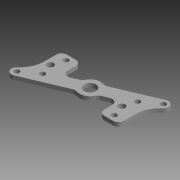
# Autodesk Inventor part: 01105
Saved by Autodesk Inventor 2015 (Build 190159000, 159)
## iProperties
Created: 2015-09-02
Part Number: 01105
Material: Generic
Description: Spring holder plate
Document SubType Name: Modeling
Designer: FC
Density: 1 g/cm^3
Appearance: Default
Part Category: 5 - Engine
Author: francis
Autodesk Inventor part; units mm, degrees
ref_plane "YZ Plane" through (0, 0, 0) normal (1, 0, 0) x (0, 1, 0)
ref_plane "XY Plane" through (0, 0, 0) normal (0, 0, 1) x (1, 0, 0)
sketch "Sketch1" plane through (0, 0, 0) normal (0, 0, 1) x (1, 0, 0)
  circle A0 centre (-10.5, 0) radius 2.067 construction
  circle A1 centre (-7.5, -9) radius 1.7295 construction
  circle A2 centre (-7.5, 9) radius 1.7295 construction
  circle A3 centre (-7.5, 9) radius 1.7295 construction
  circle A4 centre (-7.5, -9) radius 1.7295 construction
  circle A5 centre (-10.5, 0) radius 2.067 construction
  line L0 (0, -13) -> (-15, -13) construction
  line L1 (0, 13) -> (0, -13) construction
  line L2 (-15, 13) -> (0, 13) construction
  line L3 (-15, -13) -> (-15, 13) construction
  circle A6 centre (-62.5, -9) radius 1.7295 construction
  circle A7 centre (-62.5, 9) radius 1.7295 construction
  circle A8 centre (-65.5, 0) radius 2.067 construction
  line L4 (-55, -13) -> (-70, -13) construction
  line L5 (-55, 13) -> (-55, -13) construction
  line L6 (-70, 13) -> (-55, 13) construction
  line L7 (-70, -13) -> (-70, 13) construction
  spline S0 degree 3 poles (-35, 4) (-35.5054, 4) (-36.0423, 3.8984) (-37.0269, 3.4894) (-37.4748, 3.182) (-38.1819, 2.4749) (-38.4894, 2.027) (-38.8985, 1.0423) (-39, 0.5052) (-39, -0.5052) (-38.8985, -1.0423) (-38.4894, -2.027) (-38.1819, -2.4749) (-37.4748, -3.182) (-37.0269, -3.4894) (-36.0423, -3.8984) (-35.5054, -4) (-34.4946, -4) (-33.9577, -3.8984) (-32.9731, -3.4894) (-32.5252, -3.182) (-31.8181, -2.4749) (-31.5106, -2.027) (-31.1015, -1.0423) (-31, -0.5052) (-31, 0.5052) (-31.1015, 1.0423) (-31.5106, 2.027) (-31.8181, 2.4749) (-32.5252, 3.182) (-32.9731, 3.4894) (-33.9577, 3.8984) (-34.4946, 4) (-35, 4) knots 0 0 0 0 0.151609 0.151609 0.303217 0.303217 0.454789 0.454789 0.60636 0.60636 0.757932 0.757932 0.909504 0.909504 1.061112 1.061112 1.212721 1.212721 1.364329 1.364329 1.515938 1.515938 1.667509 1.667509 1.819081 1.819081 1.970653 1.970653 2.122224 2.122224 2.273833 2.273833 2.425441 2.425441 2.425441 2.425441 construction
  circle A9 centre (4, 17.3205) radius 2
  circle A10 centre (-74, -17.3205) radius 2
  line L8 (0, -9) -> (0, 0)
  line L9 (-4, -13) -> (-11, -13)
  line L10 (-59, 13) -> (-66, 13)
  line L11 (-70, 9) -> (-70, 0)
  arc A11 (-76.5934, -14.2751) -> (-72.4577, -21.0112) centre (-74, -17.3205) ccw
  arc A12 (6.5934, 14.2751) -> (2.4577, 21.0112) centre (4, 17.3205) ccw
  circle A13 centre (-10.5, 0) radius 2.5
  circle A14 centre (-7.5, -9) radius 2
  circle A15 centre (-7.5, 9) radius 2
  circle A16 centre (-65.5, 0) radius 2.5
  circle A17 centre (-62.5, -9) radius 2
  circle A18 centre (-62.5, 9) radius 2
  arc A19 (-76.5934, -14.2751) -> (-70, 0) centre (-88.75, 0) ccw
  arc A20 (6.5934, 14.2751) -> (0, 0) centre (18.75, 0) ccw
  arc A21 (-32.6046, 7.633) -> (-42.1142, 3.659) centre (-35, 0) ccw
  arc A22 (-37.3954, -7.633) -> (-27.8858, -3.659) centre (-35, 0) ccw
  arc A23 (-32.6046, 7.633) -> (-29.1796, 7.7902) centre (-31.1075, 12.4036) ccw
  line L12 (-29.1796, 7.7902) -> (2.4577, 21.0112)
  arc A24 (-37.3954, -7.633) -> (-40.8204, -7.7902) centre (-38.8925, -12.4036) ccw
  line L13 (-40.8204, -7.7902) -> (-72.4577, -21.0112)
  arc A25 (-25.3673, -1.3324) -> (-27.8858, -3.659) centre (-23.4394, -5.9458) ccw
  arc A26 (-44.6327, 1.3324) -> (-42.1142, 3.659) centre (-46.5606, 5.9458) ccw
  line L14 (-44.6327, 1.3324) -> (-49.4577, -0.6839)
  line L15 (-25.3673, -1.3324) -> (-20.5423, 0.6839)
  line L16 (-15, -3.0068) -> (-15, -9)
  line L17 (-55, 9) -> (-55, 3.0068)
  circle A27 centre (-35, 0) radius 4.5
  arc A28 (-15, -9) -> (-11, -13) centre (-11, -9) ccw
  arc A29 (-4, -13) -> (0, -9) centre (-4, -9) ccw
  arc A30 (-55, 9) -> (-59, 13) centre (-59, 9) ccw
  arc A31 (-66, 13) -> (-70, 9) centre (-66, 9) ccw
  arc A32 (-55, 3.0068) -> (-49.4577, -0.6839) centre (-51, 3.0068) ccw
  arc A33 (-15, -3.0068) -> (-20.5423, 0.6839) centre (-19, -3.0068) ccw
  line L18 (-110.25, 0) -> (40.25, 0) construction
  point P0 (-35, 4)
  point P1 (-55, -3)
  point P2 (-15, 3)
  point P3 (-55, 6.0034)
  point P4 (-7.5, -13)
  dimension "d0" = 4
  dimension "d1" = 4
  dimension "d3" = 4
  dimension "d4" = 4
  dimension "d5" = 5
  dimension "d6" = 4
  dimension "d7" = 4
  dimension "d8" = 5
  dimension "d9" = 4
  dimension "d10" = 4
  dimension "d11" = 8
  dimension "d12" = 9
  dimension "d13" = 5
  dimension "d14" = 5
  dimension "d15" = 5
  dimension "d16" = 5
  dimension "d19" = 10
  dimension "d20" = 10
  dimension "d21" = 4
  dimension "d24" = 13
  dimension "d25" = 13
  dimension "d26" = 13
  dimension "d27" = 13
  constraints: 36 end point, 33 point on circle, 26 tangent, 25 centre point, 14 point on line, 13 coincident, 5 collinear, 5 equal radius, 3 midpoint, 3 vertical, 1 horizontal alignment, 1 parallel, 1 perpendicular
  measures "d0" diameter of A9
  measures "d1" diameter of A10
  measures "d3" radius of A11
  measures "d4" radius of A12
  measures "d5" diameter of A13
  measures "d6" diameter of A14
  measures "d7" diameter of A15
  measures "d8" diameter of A16
  measures "d9" diameter of A17
  measures "d10" diameter of A18
  measures "d11" radius of A22
  measures "d12" diameter of A27
  measures "d13" distance from line of L15 A25.centre
  measures "d14" distance from line of L12 A23.centre
  measures "d15" distance from line of A24.centre L13
  measures "d16" distance from line of L14 A26.centre
  measures "d19" distance of L2.start point (-15, 3)
  measures "d20" distance of L4.start point (-55, -3)
  measures "d21" radius of A28
  measures "d24" distance between parallel lines of L4 L18
  measures "d25" distance between parallel lines of L6 L18
  measures "d26" distance between parallel lines of L2 L18
  measures "d27" distance between parallel lines of L9 L18
extrude "Extrusion1" add sketch "Sketch1" along normal blind 3
body "Solid1"
